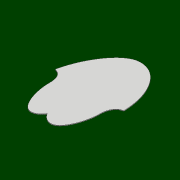
# Autodesk Inventor part: Part2
Saved by Autodesk Inventor 2018 (Build 220112000, 112)
## iProperties
Created: 2021-12-12
Part Number: Part2
Material: 一般
Document SubType Name: Modeling
Designer: gisen
Density: 1 g/cm^3
Appearance: 既定
Author: gisen
Autodesk Inventor part; units mm, degrees
ref_plane "YZ Plane" through (0, 0, 0) normal (1, 0, 0) x (0, 1, 0)
ref_plane "XZ Plane" through (0, 0, 0) normal (0, 1, 0) x (-1, 0, 0)
ref_plane "XY Plane" through (0, 0, 0) normal (0, 0, 1) x (1, 0, 0)
sketch "スケッチ1" plane through (0, 0, 0) normal (0, 0, 1) x (1, 0, 0)
  line L0 (92.5939, 154.9055) -> (93.9001, 158.0773)
  line L1 (93.9001, 158.0773) -> (95.0859, 161.3539)
  line L2 (95.0859, 161.3539) -> (96.1488, 164.7145)
  line L3 (96.1488, 164.7145) -> (97.0852, 168.138)
  line L4 (97.0852, 168.138) -> (97.8913, 171.6035)
  line L5 (97.8913, 171.6035) -> (98.5628, 175.0898)
  line L6 (98.5628, 175.0898) -> (99.095, 178.5762)
  line L7 (99.095, 178.5762) -> (99.4825, 182.0419)
  line L8 (99.4825, 182.0419) -> (99.7198, 185.4667)
  line L9 (99.7198, 185.4667) -> (99.7973, 188.6932)
  line L10 (99.7973, 188.6932) -> (99.9472, 192.1334)
  line L11 (99.9472, 192.1334) -> (100.3649, 195.2932)
  line L12 (100.3649, 195.2932) -> (101.0332, 198.2643)
  line L13 (101.0332, 198.2643) -> (101.9259, 201.0014)
  line L14 (101.9259, 201.0014) -> (103.0121, 203.4588)
  line L15 (103.0121, 203.4588) -> (104.2552, 205.5928)
  line L16 (104.2552, 205.5928) -> (105.6112, 207.3643)
  line L17 (105.6112, 207.3643) -> (107.0293, 208.7458)
  line L18 (107.0293, 208.7458) -> (108.4594, 209.7307)
  line L19 (108.4594, 209.7307) -> (110.0788, 210.4294)
  line L20 (110.0788, 210.4294) -> (114.3174, 211.7437)
  line L21 (114.3174, 211.7437) -> (114.0545, 217.0959)
  line L22 (114.0545, 217.0959) -> (113.5272, 223.0291)
  line L23 (113.5272, 223.0291) -> (112.7267, 228.8702)
  line L24 (112.7267, 228.8702) -> (111.66, 234.5851)
  line L25 (111.66, 234.5851) -> (110.3328, 240.1551)
  line L26 (110.3328, 240.1551) -> (108.7502, 245.5615)
  line L27 (108.7502, 245.5615) -> (106.9172, 250.7855)
  line L28 (106.9172, 250.7855) -> (104.8383, 255.808)
  line L29 (104.8383, 255.808) -> (102.5178, 260.6101)
  line L30 (102.5178, 260.6101) -> (99.9592, 265.1721)
  line L31 (99.9592, 265.1721) -> (97.164, 269.477)
  line L32 (97.164, 269.477) -> (94.1022, 273.533)
  line L33 (94.1022, 273.533) -> (90.8555, 277.1993)
  line L34 (90.8555, 277.1993) -> (87.4349, 280.4614)
  line L35 (87.4349, 280.4614) -> (83.8498, 283.3058)
  line L36 (83.8498, 283.3058) -> (80.1109, 285.717)
  line L37 (80.1109, 285.717) -> (76.2312, 287.6775)
  line L38 (76.2312, 287.6775) -> (72.2273, 289.1687)
  line L39 (72.2273, 289.1687) -> (68.1204, 290.1723)
  line L40 (68.1204, 290.1723) -> (63.9359, 290.6719)
  line L41 (63.9359, 290.6719) -> (59.8151, 290.6558)
  line L42 (59.8151, 290.6558) -> (59.4481, 290.63)
  line L43 (59.4481, 290.63) -> (59.1858, 290.6082)
  line L44 (59.1858, 290.6082) -> (58.922, 290.5831)
  line L45 (58.922, 290.5831) -> (58.6568, 290.5546)
  line L46 (58.6568, 290.5546) -> (58.3902, 290.5228)
  line L47 (58.3902, 290.5228) -> (58.1226, 290.4878)
  line L48 (58.1226, 290.4878) -> (57.854, 290.4498)
  line L49 (57.854, 290.4498) -> (57.5839, 290.4085)
  line L50 (57.5839, 290.4085) -> (57.3127, 290.3641)
  line L51 (57.3127, 290.3641) -> (56.9195, 290.2956)
  line L52 (56.9195, 290.2956) -> (53.8145, 289.5232)
  line L53 (53.8145, 289.5232) -> (50.6093, 288.3027)
  line L54 (50.6093, 288.3027) -> (47.4335, 286.6929)
  line L55 (47.4335, 286.6929) -> (44.2888, 284.7153)
  line L56 (44.2888, 284.7153) -> (41.1758, 282.3863)
  line L57 (41.1758, 282.3863) -> (38.0964, 279.7186)
  line L58 (38.0964, 279.7186) -> (35.054, 276.7229)
  line L59 (35.054, 276.7229) -> (32.0534, 273.4087)
  line L60 (32.0534, 273.4087) -> (29.1007, 269.7844)
  line L61 (29.1007, 269.7844) -> (26.204, 265.8597)
  line L62 (26.204, 265.8597) -> (23.4596, 261.7806)
  line L63 (23.4596, 261.7806) -> (20.8421, 257.5279)
  line L64 (20.8421, 257.5279) -> (18.3572, 253.1172)
  line L65 (18.3572, 253.1172) -> (16.0116, 248.5654)
  line L66 (16.0116, 248.5654) -> (13.8123, 243.8894)
  line L67 (13.8123, 243.8894) -> (11.7664, 239.1061)
  line L68 (11.7664, 239.1061) -> (9.8813, 234.2323)
  line L69 (9.8813, 234.2323) -> (8.1647, 229.2846)
  line L70 (8.1647, 229.2846) -> (6.6243, 224.2798)
  line L71 (6.6243, 224.2798) -> (5.2776, 219.2707)
  line L72 (5.2776, 219.2707) -> (4.0555, 214.3719)
  line L73 (4.0555, 214.3719) -> (8.5234, 212.3603)
  line L74 (8.5234, 212.3603) -> (9.8405, 211.6758)
  line L75 (9.8405, 211.6758) -> (11.0799, 210.833)
  line L76 (11.0799, 210.833) -> (12.3101, 209.7467)
  line L77 (12.3101, 209.7467) -> (13.5094, 208.3691)
  line L78 (13.5094, 208.3691) -> (14.6515, 206.6435)
  line L79 (14.6515, 206.6435) -> (15.701, 204.5087)
  line L80 (15.701, 204.5087) -> (16.6125, 201.9046)
  line L81 (16.6125, 201.9046) -> (17.3333, 198.777)
  line L82 (17.3333, 198.777) -> (17.8072, 195.0787)
  line L83 (17.8072, 195.0787) -> (17.9826, 190.6474)
  line L84 (17.9826, 190.6474) -> (18.0567, 187.4174)
  line L85 (18.0567, 187.4174) -> (18.2821, 183.971)
  line L86 (18.2821, 183.971) -> (18.6487, 180.4607)
  line L87 (18.6487, 180.4607) -> (19.15, 176.9121)
  line L88 (19.15, 176.9121) -> (19.7801, 173.3513)
  line L89 (19.7801, 173.3513) -> (20.5335, 169.8045)
  line L90 (20.5335, 169.8045) -> (21.4052, 166.2985)
  line L91 (21.4052, 166.2985) -> (22.3907, 162.8598)
  line L92 (22.3907, 162.8598) -> (23.486, 159.5147)
  line L93 (23.486, 159.5147) -> (24.6885, 156.2878)
  line L94 (24.6885, 156.2878) -> (26.026, 153.1412)
  line L95 (26.026, 153.1412) -> (27.4395, 150.2378)
  line L96 (27.4395, 150.2378) -> (28.9253, 147.5866)
  line L97 (28.9253, 147.5866) -> (30.484, 145.1942)
  line L98 (30.484, 145.1942) -> (32.1223, 143.067)
  line L99 (32.1223, 143.067) -> (33.8558, 141.2129)
  line L100 (33.8558, 141.2129) -> (35.7122, 139.6474)
  line L101 (35.7122, 139.6474) -> (37.7317, 138.406)
  line L102 (37.7317, 138.406) -> (39.9493, 137.566)
  line L103 (39.9493, 137.566) -> (42.2174, 137.2701)
  line L104 (42.2174, 137.2701) -> (44.4372, 137.433)
  line L105 (44.4372, 137.433) -> (46.4952, 137.888)
  line L106 (46.4952, 137.888) -> (48.4765, 138.6234)
  line L107 (48.4765, 138.6234) -> (50.3637, 139.615)
  line L108 (50.3637, 139.615) -> (52.149, 140.8395)
  line L109 (52.149, 140.8395) -> (53.8311, 142.2776)
  line L110 (53.8311, 142.2776) -> (55.4121, 143.9146)
  line L111 (55.4121, 143.9146) -> (56.8952, 145.7401)
  line L112 (56.8952, 145.7401) -> (58.1851, 147.6048)
  line L113 (58.1851, 147.6048) -> (58.7984, 146.6239)
  line L114 (58.7984, 146.6239) -> (60.3519, 144.5257)
  line L115 (60.3519, 144.5257) -> (62.021, 142.6395)
  line L116 (62.021, 142.6395) -> (63.8076, 140.9772)
  line L117 (63.8076, 140.9772) -> (65.7139, 139.5557)
  line L118 (65.7139, 139.5557) -> (67.74, 138.3974)
  line L119 (67.74, 138.3974) -> (69.8795, 137.5313)
  line L120 (69.8795, 137.5313) -> (72.1148, 136.9903)
  line L121 (72.1148, 136.9903) -> (74.482, 136.7992)
  line L122 (74.482, 136.7992) -> (76.7622, 137.0637)
  line L123 (76.7622, 137.0637) -> (78.9909, 137.821)
  line L124 (78.9909, 137.821) -> (81.0578, 138.9687)
  line L125 (81.0578, 138.9687) -> (82.9788, 140.4402)
  line L126 (82.9788, 140.4402) -> (84.7817, 142.1992)
  line L127 (84.7817, 142.1992) -> (86.4902, 144.2283)
  line L128 (86.4902, 144.2283) -> (88.1199, 146.5186)
  line L129 (88.1199, 146.5186) -> (89.6789, 149.0648)
  line L130 (89.6789, 149.0648) -> (91.1704, 151.862)
  line L131 (91.1704, 151.862) -> (92.5939, 154.9055)
  constraints: 264 end point
extrude "押し出し1" add sketch "スケッチ1" along normal blind 1
